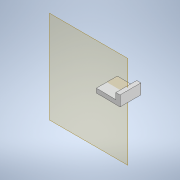
# Autodesk Inventor part: gira  down
Saved by Autodesk Inventor 2020 (Build 240168000, 168)
## iProperties
Created: 2023-03-26
Part Number: gira  down
Material: Generic
Document SubType Name: Modeling
Designer: super
Density: 1 g/cm^3
Appearance: Default
Author: super
Autodesk Inventor part; units mm, degrees
ref_plane "YZ Plane" through (0, 0, 0) normal (1, 0, 0) x (0, 1, 0)
ref_plane "XZ Plane" through (0, 0, 0) normal (0, 1, 0) x (-1, 0, 0)
ref_plane "XY Plane" through (0, 0, 0) normal (0, 0, 1) x (1, 0, 0)
ref_plane "Work Plane1" through (0, 200, 0) normal (0, 0, 1) x (-1, 0, 0)
sketch "Sketch1" plane through (0, 200, 0) normal (0, 0, 1) x (-1, 0, 0)
  line L0 (-15.0122, 49.9064) -> (-15.0122, 74.6271)
  line L1 (-15.0122, 74.6271) -> (41.5559, 74.0451)
  line L2 (41.5559, 64.0446) -> (-5.0122, 64.5237)
  line L3 (-5.0122, 64.5237) -> (-5.0122, 49.9064)
  line L4 (-15.0122, 49.9064) -> (-5.0122, 49.9064)
  line L5 (41.5559, 64.0446) -> (41.5559, 74.0451)
  point P0 (0, 200)
  dimension "d1" = 10
  constraints: 12 end point, 1 horizontal, 1 perpendicular, 1 vertical, 1 other
  measures "d1" distance between parallel lines of L1 L2
extrude "Extrusion1" add sketch "Sketch1" along normal mid plane 50
body "Solid1"
